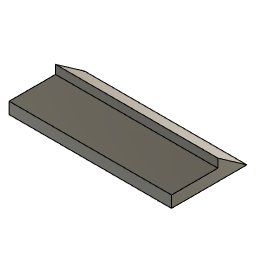
AttacheUpIns v2 (Autodesk Fusion 360 design; units mm, degrees)
Autodesk Fusion 360 part; units mm, degrees
sketch "Esquisse1" plane through (0, 0, 0) normal (0, 0, 1) x (1, 0, 0)
  line L0 (0, 0) -> (28, 0)
  line L1 (28, 0) -> (28, 13)
  line L2 (28, 13) -> (0, 13)
  line L3 (0, 13) -> (0, 0)
  dimension "d1" = 28
  dimension "d2" = 13
  constraint horizontal L0
  constraint vertical L1
  constraint horizontal L2
  constraint vertical L3
  constraint coincident L0.start L3.end
  measures "d1" distance of L1.end L2.end
  measures "d2" distance of L0.end L1.end
extrude "Extrusion1" add sketch "Esquisse1" along normal blind 2
sketch "Esquisse2" plane through (0, 0, 2) normal (0, 0, 1) x (-1, 0, 0)
  line L0 (0, -13) -> (0, 0)
  line L1 (0, 0) -> (-28, 0)
  line L2 (-28, 0) -> (-28, -13)
  line L3 (-28, -13) -> (0, -13)
  line L4 (0, -13) -> (-28, -13)
  line L5 (-28, -13) -> (-28, -8)
  line L6 (-28, -8) -> (0, -8)
  line L7 (0, -8) -> (0, -13)
  dimension "d5" = 5
  constraint horizontal L4
  constraint vertical L5
  constraint horizontal L6
  constraint vertical L7
  constraint coincident L2 L5.end
  constraint coincident L0.start L3.end
  measures "d5" distance of L2.end L5.end
extrude "Extrusion2" add sketch "Esquisse2" along normal blind 1.5 contours L0 L2 L3 L4 L5 L6 L7
chamfer "Chanfrein1" distance 5 distance2 3.5 1 edges at (14, 13, 3.5) measured on face at (9.3333, 11.3333, 3.5)
